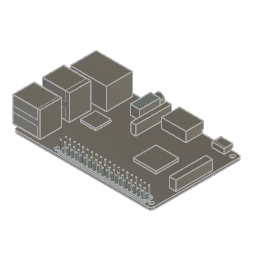
my.mesh_Gehäuse (Autodesk Fusion 360 archive; units mm, degrees)
design "Raspberry_Pi_3_B"
Autodesk Fusion 360 part; units mm, degrees
sketch "Sketch1" plane through (0, 0, 0) normal (0, 0, 1) x (1, 0, 0) in component "Pi"
  line L0 (42.5, 28) -> (-42.5, 28)
  line L1 (-42.5, 28) -> (-42.5, -28)
  line L2 (-42.5, -28) -> (42.5, -28)
  line L3 (42.5, -28) -> (42.5, 28)
  line L4 (42.5, 28) -> (-42.5, -28) construction
  line L5 (-42.5, 28) -> (42.5, -28) construction
  dimension "d1" = 85
  dimension "d2" = 56
  constraint perpendicular L0 L1
  constraint parallel L0 L2
  constraint parallel L1 L3
  constraint horizontal L0
  constraint coincident L4 origin
  constraint coincident L5 origin
  measures "d1" distance of L1.end L2.end
  measures "d2" distance of L0.end L1.end
extrude "Extrude1" add sketch "Sketch1" along normal blind 1.4 makes body 1 in component "Pi"
fillet "Fillet1" radius 2 4 edges at (42.5, -28, 0.7) (42.5, 28, 0.7) (-42.5, 28, 0.7) (-42.5, -28, 0.7) on bodies 1 in component "Pi"
sketch "Sketch2" plane through (0, 0, 1.4) normal (0, 0, 1) x (-1, 0, 0) in component "Pi"
  arc A0 (42.5, 26) -> (40.5, 28) centre (40.5, 26) ccw
  line L0 (40.5, 28) -> (-40.5, 28)
  arc A1 (-40.5, 28) -> (-42.5, 26) centre (-40.5, 26) ccw
  line L1 (-42.5, 26) -> (-42.5, -26)
  arc A2 (-42.5, -26) -> (-40.5, -28) centre (-40.5, -26) ccw
  line L2 (-40.5, -28) -> (40.5, -28)
  arc A3 (40.5, -28) -> (42.5, -26) centre (40.5, -26) ccw
  line L3 (42.5, -26) -> (42.5, 26)
  line L4 (42.5, -24.7968) -> (23.2, -24.7968) construction
  line L5 (23.2, -28) -> (23.2, -26) construction
  line L6 (23.2, -26) -> (45.5, -26)
  line L7 (45.5, -26) -> (45.5, -10)
  line L8 (45.5, -10) -> (23.2, -10)
  line L9 (23.2, -10) -> (23.2, -26)
  dimension "d6" = 19.3
  dimension "d7" = 22.3
  dimension "d8" = 16
  constraint coincident L3 L4.start
  constraint perpendicular L3 L4
  constraint coincident L2 L5.start
  constraint perpendicular L2 L5
  constraint horizontal L6
  constraint vertical L7
  constraint horizontal L8
  constraint vertical L9
  measures "d6" distance of L4.start L4.end
  measures "d7" distance of L5.end L6.end
  measures "d8" distance of L5.end L8.end
extrude "Extrude2" add sketch "Sketch2" along normal blind 13.5 contours L3 L6 L7 L8 | L3 L6 L8 L9 bodies 1 in component "Pi"
copy_body "CutPasteBodies1" bodies 1 removing the originals makes body 2 in component "Pi"
sketch "Sketch1 (1)" plane through (0, 0, 1.4) normal (0, 0, 1) x (-1, 0, 0) in component "Pi"
  line L0 (23.2, -10) -> (42.5, -10)
  line L1 (42.5, -10) -> (42.5, 26)
  arc A0 (42.5, 26) -> (40.5, 28) centre (40.5, 26) ccw
  line L2 (40.5, 28) -> (-40.5, 28)
  arc A1 (-40.5, 28) -> (-42.5, 26) centre (-40.5, 26) ccw
  line L3 (-42.5, 26) -> (-42.5, -26)
  arc A2 (-42.5, -26) -> (-40.5, -28) centre (-40.5, -26) ccw
  line L4 (-40.5, -28) -> (40.5, -28)
  arc A3 (40.5, -28) -> (42.5, -26) centre (40.5, -26) ccw
  line L5 (42.5, -26) -> (23.2, -26)
  line L6 (23.2, -26) -> (23.2, -10)
  line L7 (36, -10) -> (36, -6) construction
  line L8 (-41.9142, -27.4142) -> (-39.5808, -25.0808)
  line L9 (-41.9142, -27.4142) -> (-38.6142, -27.4142) construction
  circle A4 centre (-39.5808, -25.0808) radius 1.3
  dimension "d46" = 3.3
  dimension "d47" = 45
  dimension "d48" = 2.6
  constraint parallel L1 L7
  constraint midpoint A2 L8.start
  constraint horizontal L9
  constraint coincident L8.end A4.centre
  measures "d46" distance of L8.start L8.end
  measures "d47" angle of L8 L9
  measures "d48" diameter of A4
sketch "Sketch2 (1)" plane through (-45.5, 0, 0) normal (-1, 0, 0) x (0, -1, 0) in component "Pi"
  line L0 (-26, 1.4) -> (-10, 1.4)
  line L1 (-10, 1.4) -> (-10, 14.9)
  line L2 (-10, 14.9) -> (-26, 14.9)
  line L3 (-26, 14.9) -> (-26, 1.4)
  line L4 (-6, 1.4) -> (7.2, 1.4)
  line L5 (7.2, 1.4) -> (7.2, 17.15)
  line L6 (7.2, 17.15) -> (-6, 17.15)
  line L7 (-6, 17.15) -> (-6, 1.4)
  point P0 (-6, 1.4)
  dimension "d11" = 13.2
  dimension "d12" = 15.75
  constraint horizontal L4
  constraint vertical L5
  constraint horizontal L6
  constraint vertical L7
  constraint coincident P0 L4.start
  measures "d11" distance of P0 L4.end
  measures "d12" distance of P0 L6.end
extrude "Extrude1'" add sketch "Sketch2 (1)" against normal blind 16.7 contours L4 L5 L6 L7 bodies 2 in component "Pi"
sketch "Sketch3" plane through (-45.5, 0, 0) normal (-1, 0, 0) x (0, -1, 0) in component "Pi"
  line L0 (-6, 17.15) -> (-6, 1.4)
  line L1 (-6, 1.4) -> (7.2, 1.4)
  line L2 (7.2, 1.4) -> (7.2, 17.15)
  line L3 (7.2, 17.15) -> (-6, 17.15)
  line L4 (7.2, 1.4) -> (12.2, 1.4) construction
  line L5 (12.2, 1.4) -> (25.4, 1.4)
  line L6 (25.4, 1.4) -> (25.4, 17.15)
  line L7 (25.4, 17.15) -> (12.2, 17.15)
  line L8 (12.2, 17.15) -> (12.2, 1.4)
  dimension "d15" = 5
  dimension "d16" = 13.2
  dimension "d17" = 15.75
  constraint coincident L1.end L2.start
  constraint perpendicular L2 L4
  constraint horizontal L5
  constraint vertical L6
  constraint horizontal L7
  constraint vertical L8
  measures "d15" distance of L1.end L4.end
  measures "d16" distance of L4.end L5.end
  measures "d17" distance of L4.end L7.end
extrude "Extrude2'" add sketch "Sketch3" against normal blind 16.75 contours L5 L6 L7 L8 bodies 2 in component "Pi"
sketch "Sketch4" plane through (-45.5, 0, 0) normal (-1, 0, 0) x (0, -1, 0) in component "Pi"
  line L0 (-26, 1.4) -> (-10, 1.4)
  line L1 (-10, 1.4) -> (-10, 14.9)
  line L2 (-10, 14.9) -> (-26, 14.9)
  line L3 (-26, 14.9) -> (-26, 1.4)
  line L4 (-20.2136, 14.9) -> (-20.2136, 12.2) construction
  line L5 (-26, 12.2) -> (-24, 12.2) construction
  line L6 (-24, 12.2) -> (-12, 12.2)
  line L7 (-12, 12.2) -> (-12, 5.5)
  line L8 (-12, 5.5) -> (-24, 5.5)
  line L9 (-24, 5.5) -> (-24, 12.2)
  line L10 (-26, 5.5) -> (-21.25, 5.5) construction
  line L11 (-21.25, 5.5) -> (-15.25, 5.5)
  line L12 (-15.25, 5.5) -> (-15.25, 2)
  line L13 (-15.25, 2) -> (-21.25, 2)
  line L14 (-21.25, 2) -> (-21.25, 5.5)
  dimension "d20" = 2.7
  dimension "d21" = 12
  dimension "d22" = 6.7
  dimension "d23" = 4.75
  dimension "d24" = 6
  dimension "d25" = 3.5
  constraint coincident L2 L4.start
  constraint perpendicular L2 L4
  constraint coincident L3 L5.start
  constraint perpendicular L3 L5
  constraint horizontal L6
  constraint vertical L7
  constraint horizontal L8
  constraint vertical L9
  constraint coincident L3 L10.start
  constraint perpendicular L3 L10
  constraint horizontal L11
  constraint vertical L12
  constraint horizontal L13
  constraint vertical L14
  constraint coincident L8 L11.end
  measures "d20" distance of L4.start L4.end
  measures "d21" distance of L5.end L6.end
  measures "d22" distance of L5.end L8.end
  measures "d23" distance of L10.start L10.end
  measures "d24" distance of L10.end L11.end
  measures "d25" distance of L10.end L13.end
extrude "Extrude3" cut sketch "Sketch4" against normal blind 17 contours L6 L7 L8 L9 L11 | L8 L11 L12 L13 L14 bodies 2 in component "Pi"
sketch "Sketch5" plane through (-45.5, 0, 0) normal (-1, 0, 0) x (0, -1, 0) in component "Pi"
  line L0 (-6, 17.15) -> (-6, 1.4)
  line L1 (-6, 1.4) -> (7.2, 1.4)
  line L2 (7.2, 1.4) -> (7.2, 17.15)
  line L3 (7.2, 17.15) -> (-6, 17.15)
  line L4 (7.2, 10.975) -> (-6, 10.975)
  line L5 (-6, 10.975) -> (-6, 7.575)
  line L6 (-6, 7.575) -> (7.2, 7.575)
  line L7 (7.2, 7.575) -> (7.2, 10.975)
  line L8 (7.2, 10.975) -> (-6, 7.575) construction
  line L9 (-6, 10.975) -> (7.2, 7.575) construction
  line L10 (-5.7208, 10.975) -> (6.8067, 10.975)
  line L11 (6.8067, 10.975) -> (6.8067, 16.8566)
  line L12 (6.8067, 16.8566) -> (-5.7208, 16.8566)
  line L13 (-5.7208, 16.8566) -> (-5.7208, 10.975)
  line L14 (-5.7208, 7.6469) -> (6.8067, 7.6469)
  line L15 (6.8067, 7.6469) -> (6.8067, 1.6277)
  line L16 (6.8067, 1.6277) -> (-5.7208, 1.6277)
  line L17 (-5.7208, 1.6277) -> (-5.7208, 7.6469)
  point P0 (0.6, 9.275)
  dimension "d28" = 3.4
  constraint perpendicular L4 L5
  constraint parallel L4 L6
  constraint parallel L5 L7
  constraint horizontal L4
  constraint coincident L8 P0
  constraint coincident L9 P0
  constraint horizontal L10
  constraint vertical L11
  constraint horizontal L12
  constraint vertical L13
  constraint coincident L4 L10.start
  constraint horizontal L14
  constraint vertical L15
  constraint horizontal L16
  constraint vertical L17
  constraint coincident L8 L14.start
  measures "d28" distance of L4.end L5.end
extrude "Extrude4" cut sketch "Sketch5" against normal blind 14 contours L4 L10 L11 L12 L13 | L6 L15 L16 L17 bodies 2 in component "Pi"
sketch "Sketch6" plane through (-45.5, 0, 0) normal (-1, 0, 0) x (0, -1, 0) in component "Pi"
  line L0 (12.2, 17.15) -> (12.2, 1.4)
  line L1 (12.2, 1.4) -> (25.4, 1.4)
  line L2 (25.4, 1.4) -> (25.4, 17.15)
  line L3 (25.4, 17.15) -> (12.2, 17.15)
  line L4 (12.4971, 16.7794) -> (25.17, 16.7794)
  line L5 (25.17, 16.7794) -> (25.17, 10.9805)
  line L6 (25.17, 10.9805) -> (12.4971, 10.9805)
  line L7 (12.4971, 10.9805) -> (12.4971, 16.7794)
  line L8 (12.4971, 7.5659) -> (25.17, 7.5659)
  line L9 (25.17, 7.5659) -> (25.17, 1.5998)
  line L10 (25.17, 1.5998) -> (12.4971, 1.5998)
  line L11 (12.4971, 1.5998) -> (12.4971, 7.5659)
  constraint horizontal L4
  constraint vertical L5
  constraint horizontal L6
  constraint vertical L7
  constraint horizontal L8
  constraint vertical L9
  constraint horizontal L10
  constraint vertical L11
extrude "Extrude5" cut sketch "Sketch6" against normal blind 15 contours L4 L5 L6 L7 | L8 L9 L10 L11 bodies 2 in component "Pi"
sketch "Sketch7" plane through (0, 28, 0) normal (0, 1, 0) x (-1, 0, 0) in component "Pi"
  line L0 (40.5, 0) -> (40.5, 1.4)
  line L1 (40.5, 1.4) -> (-40.5, 1.4)
  line L2 (-40.5, 1.4) -> (-40.5, 0)
  line L3 (-40.5, 0) -> (40.5, 0)
  line L4 (42.5, 1.4) -> (42.5, 0)
  line L5 (42.5, 0.7) -> (11, 0.7) construction
  circle A0 centre (11.0002, 4.35) radius 2.95
  dimension "d33" = 31.5
  dimension "d34" = 5.9
  constraint midpoint L4 L5.start
  constraint perpendicular L0 L5
  measures "d33" distance of L5.start L5.end
  measures "d34" diameter of A0
extrude "Extrude6" add sketch "Sketch7" along normal blind 3 separate body contours A0 makes body 3 in component "Pi"
sketch "Sketch8" plane through (0, 28, 0) normal (0, -1, 0) x (1, 0, 0) in component "Pi"
  arc A0 (-10.9892, 1.4) -> (-11.0112, 1.4) centre (-11.0002, 4.35) ccw
  line L0 (-11.0112, 1.4) -> (-10.9892, 1.4)
  line L1 (-8.0502, 7.3) -> (-13.9502, 7.3)
  line L2 (-13.9502, 7.3) -> (-13.9502, 1.4)
  line L3 (-13.9502, 1.4) -> (-8.0502, 1.4)
  line L4 (-8.0502, 1.4) -> (-8.0502, 7.3)
  line L5 (-8.0502, 7.3) -> (-13.9502, 1.4) construction
  line L6 (-13.9502, 7.3) -> (-8.0502, 1.4) construction
  point P0 (-11.0002, 4.35)
  dimension "d37" = 5.9
  constraint perpendicular L1 L2
  constraint parallel L1 L3
  constraint parallel L2 L4
  constraint horizontal L1
  constraint coincident L5 P0
  constraint coincident L6 P0
  constraint coincident P0 A0.centre
  measures "d37" distance of L2.end L3.end
extrude "Extrude7" add sketch "Sketch8" along normal blind 12.5 bodies 2 3 in component "Pi"
ref_plane "WorkPlane1" through (0, 0, 1.4) normal (0, 0, 1) x (-1, 0, 0) in component "Pi"
sketch "Sketch9" plane through (0, 0, 1.4) normal (0, 0, 1) x (1, 0, 0) in component "Pi"
  line L0 (-13.9502, 15.5) -> (-13.9502, 28)
  line L1 (-28.8, 6) -> (-25.8, 6) construction
  line L2 (-25.8, 6) -> (-16.3, 6)
  line L3 (-16.3, 6) -> (-16.3, -3.5)
  line L4 (-16.3, -3.5) -> (-25.8, -3.5)
  line L5 (-25.8, -3.5) -> (-25.8, 6)
  point P0 (-28.8, 6)
  dimension "d41" = 3
  dimension "d42" = 9.5
  dimension "d43" = 9.5
  constraint coincident P0 L1.start
  constraint perpendicular L0 L1
  constraint horizontal L2
  constraint vertical L3
  constraint horizontal L4
  constraint vertical L5
  measures "d41" distance of P0 L1.end
  measures "d42" distance of L1.end L4.end
  measures "d43" distance of L1.end L2.end
extrude "Extrude8" add sketch "Sketch9" along normal blind 1.2 bodies 2 in component "Pi"
extrude "Extrude9" cut sketch "Sketch1 (1)" against normal up to surface (1.4 mm away) contours A4 bodies 2 in component "Pi"
mirror "Mirror1" about plane through (0, 0, 0) normal (0, 1, 0) of "Extrude9" in component "Pi"
sketch "Sketch10" plane through (0, 0, 1.4) normal (0, 0, 1) x (-1, 0, 0) in component "Pi"
  circle A0 centre (-39.5808, 25.0808) radius 1.3
  circle A1 centre (-39.5808, -25.0808) radius 1.3
  line L0 (25.8, 3.5) -> (25.8, -6)
  line L1 (25.8, -6) -> (16.3, -6)
  line L2 (16.3, -6) -> (16.3, 3.5)
  line L3 (16.3, 3.5) -> (25.8, 3.5)
  line L4 (13.9502, -15.5) -> (13.9502, -28)
  line L5 (13.9502, -28) -> (40.5, -28)
  arc A2 (40.5, -28) -> (42.5, -26) centre (40.5, -26) ccw
  line L6 (42.5, -26) -> (23.2, -26)
  line L7 (23.2, -26) -> (23.2, -10)
  line L8 (23.2, -10) -> (42.5, -10)
  line L9 (42.5, -10) -> (42.5, -6)
  line L10 (42.5, -6) -> (28.8, -6)
  line L11 (28.8, -6) -> (28.8, 7.2)
  line L12 (28.8, 7.2) -> (42.5, 7.2)
  line L13 (42.5, 7.2) -> (42.5, 12.2)
  line L14 (42.5, 12.2) -> (28.75, 12.2)
  line L15 (28.75, 12.2) -> (28.75, 25.4)
  line L16 (28.75, 25.4) -> (42.5, 25.4)
  line L17 (42.5, 25.4) -> (42.5, 26)
  arc A3 (42.5, 26) -> (40.5, 28) centre (40.5, 26) ccw
  line L18 (40.5, 28) -> (-40.5, 28)
  arc A4 (-40.5, 28) -> (-42.5, 26) centre (-40.5, 26) ccw
  line L19 (-42.5, 26) -> (-42.5, -26)
  arc A5 (-42.5, -26) -> (-40.5, -28) centre (-40.5, -26) ccw
  line L20 (-40.5, -28) -> (8.0502, -28)
  line L21 (8.0502, -28) -> (8.0502, -15.5)
  line L22 (8.0502, -15.5) -> (13.9502, -15.5)
  line L23 (-39.5808, 25.0808) -> (18.4192, 25.0808) construction
  circle A6 centre (18.4192, 25.0808) radius 1.35
  dimension "d52" = 58
  dimension "d53" = 2.7
  constraint coincident A0.centre L23.start
  constraint horizontal L23
  constraint coincident L23.end A6.centre
  measures "d52" distance of A0.centre L23.end
  measures "d53" diameter of A6
extrude "Extrude10" cut sketch "Sketch10" against normal up to surface (1.4 mm away) contours A6 bodies 2 in component "Pi"
mirror "Mirror2" about plane through (0, 0, 0) normal (0, 1, 0) of "Extrude10" in component "Pi"
sketch "Sketch11" plane through (0, 0, 1.4) normal (0, 0, 1) x (-1, 0, 0) in component "Pi"
  circle A0 centre (18.4192, -25.0808) radius 1.35
  circle A1 centre (18.4192, 25.0808) radius 1.35
  circle A2 centre (-39.5808, 25.0808) radius 1.3
  circle A3 centre (-39.5808, -25.0808) radius 1.3
  line L0 (25.8, 3.5) -> (25.8, -6)
  line L1 (25.8, -6) -> (16.3, -6)
  line L2 (16.3, -6) -> (16.3, 3.5)
  line L3 (16.3, 3.5) -> (25.8, 3.5)
  line L4 (13.9502, -15.5) -> (13.9502, -28)
  line L5 (13.9502, -28) -> (40.5, -28)
  arc A4 (40.5, -28) -> (42.5, -26) centre (40.5, -26) ccw
  line L6 (42.5, -26) -> (23.2, -26)
  line L7 (23.2, -26) -> (23.2, -10)
  line L8 (23.2, -10) -> (42.5, -10)
  line L9 (42.5, -10) -> (42.5, -6)
  line L10 (42.5, -6) -> (28.8, -6)
  line L11 (28.8, -6) -> (28.8, 7.2)
  line L12 (28.8, 7.2) -> (42.5, 7.2)
  line L13 (42.5, 7.2) -> (42.5, 12.2)
  line L14 (42.5, 12.2) -> (28.75, 12.2)
  line L15 (28.75, 12.2) -> (28.75, 25.4)
  line L16 (28.75, 25.4) -> (42.5, 25.4)
  line L17 (42.5, 25.4) -> (42.5, 26)
  arc A5 (42.5, 26) -> (40.5, 28) centre (40.5, 26) ccw
  line L18 (40.5, 28) -> (-40.5, 28)
  arc A6 (-40.5, 28) -> (-42.5, 26) centre (-40.5, 26) ccw
  line L19 (-42.5, 26) -> (-42.5, -26)
  arc A7 (-42.5, -26) -> (-40.5, -28) centre (-40.5, -26) ccw
  line L20 (-40.5, -28) -> (8.0502, -28)
  line L21 (8.0502, -28) -> (8.0502, -15.5)
  line L22 (8.0502, -15.5) -> (13.9502, -15.5)
  line L23 (16, 27) -> (-37.4592, 27)
  line L24 (-37.4592, 27) -> (-37.4592, 22)
  line L25 (-37.4592, 22) -> (16, 22)
  line L26 (16, 22) -> (16, 27)
  dimension "d57" = 5
  constraint horizontal L23
  constraint vertical L24
  constraint horizontal L25
  constraint vertical L26
  measures "d57" distance of L23.start L25.end
extrude "Extrude11" add sketch "Sketch11" along normal blind 1 contours L23 L24 L25 L26 bodies 2 in component "Pi"
sketch "Sketch12" plane through (0, 0, 2.4) normal (0, 0, 1) x (-1, 0, 0) in component "Pi"
  line L0 (16, 22) -> (16, 27)
  line L1 (16, 27) -> (-37.4592, 27)
  line L2 (-37.4592, 27) -> (-37.4592, 22)
  line L3 (-37.4592, 22) -> (16, 22)
  circle A0 centre (15.2841, 26.0134) radius 0.375
  dimension "d60" = 0.75
  measures "d60" diameter of A0
extrude "Extrude12" add sketch "Sketch12" along normal blind 6 contours A0 bodies 2 in component "Pi"
sketch "Sketch13" plane through (0, 0, 2.4) normal (0, 0, 1) x (-1, 0, 0) in component "Pi"
  circle A0 centre (15.2841, 26.0134) radius 0.375
  line L0 (16, 22) -> (16, 27)
  line L1 (16, 27) -> (-37.4592, 27)
  line L2 (-37.4592, 27) -> (-37.4592, 22)
  line L3 (-37.4592, 22) -> (16, 22)
ref_plane "WorkPlane2" through (10.7296, -24.5, 1.9) normal (0, -1, 0) x (1, 0, 0) in component "Pi"
mirror "Mirror3" about plane through (10.7296, -24.5, 1.9) normal (0, -1, 0) of "Extrude12" in component "Pi"
pattern_path "PathPattern2" count 20 spacing 2.7174 from (-16, -22, 1.4) along 1 edges at (10.7296, -22, 1.4) of "Extrude12", "Mirror3" on bodies 2 in component "Pi"
sketch "Sketch14" plane through (0, 0, 1.4) normal (0, 0, 1) x (-1, 0, 0) in component "Pi"
  line L0 (16, 22) -> (-37.4592, 22)
  line L1 (-37.4592, 22) -> (-37.4592, 27)
  line L2 (-37.4592, 27) -> (16, 27)
  line L3 (16, 27) -> (16, 22)
  circle A0 centre (18.4192, -25.0808) radius 1.35
  circle A1 centre (18.4192, 25.0808) radius 1.35
  circle A2 centre (-39.5808, 25.0808) radius 1.3
  circle A3 centre (-39.5808, -25.0808) radius 1.3
  line L4 (25.8, 3.5) -> (25.8, -6)
  line L5 (25.8, -6) -> (16.3, -6)
  line L6 (16.3, -6) -> (16.3, 3.5)
  line L7 (16.3, 3.5) -> (25.8, 3.5)
  line L8 (13.9502, -15.5) -> (13.9502, -28)
  line L9 (13.9502, -28) -> (40.5, -28)
  arc A4 (40.5, -28) -> (42.5, -26) centre (40.5, -26) ccw
  line L10 (42.5, -26) -> (23.2, -26)
  line L11 (23.2, -26) -> (23.2, -10)
  line L12 (23.2, -10) -> (42.5, -10)
  line L13 (42.5, -10) -> (42.5, -6)
  line L14 (42.5, -6) -> (28.8, -6)
  line L15 (28.8, -6) -> (28.8, 7.2)
  line L16 (28.8, 7.2) -> (42.5, 7.2)
  line L17 (42.5, 7.2) -> (42.5, 12.2)
  line L18 (42.5, 12.2) -> (28.75, 12.2)
  line L19 (28.75, 12.2) -> (28.75, 25.4)
  line L20 (28.75, 25.4) -> (42.5, 25.4)
  line L21 (42.5, 25.4) -> (42.5, 26)
  arc A5 (42.5, 26) -> (40.5, 28) centre (40.5, 26) ccw
  line L22 (40.5, 28) -> (-40.5, 28)
  arc A6 (-40.5, 28) -> (-42.5, 26) centre (-40.5, 26) ccw
  line L23 (-42.5, 26) -> (-42.5, -26)
  arc A7 (-42.5, -26) -> (-40.5, -28) centre (-40.5, -26) ccw
  line L24 (-40.5, -28) -> (8.0502, -28)
  line L25 (8.0502, -28) -> (8.0502, -15.5)
  line L26 (8.0502, -15.5) -> (13.9502, -15.5)
  line L27 (-42.5, 28.0113) -> (-25.5, 28.0113) construction
  line L28 (-25.5, 28.0113) -> (-25.5, 8.0113) construction
  line L29 (-25.5, 8.0113) -> (-42.5, 8.0113) construction
  line L30 (-42.5, 8.0113) -> (-42.5, 28.0113) construction
  line L31 (-25.5, 8.0113) -> (-11.5, 8.0113)
  line L32 (-11.5, 8.0113) -> (-11.5, -5.9887)
  line L33 (-11.5, -5.9887) -> (-25.5, -5.9887)
  line L34 (-25.5, -5.9887) -> (-25.5, 8.0113)
  dimension "d69" = 17
  dimension "d70" = 20
  dimension "d71" = 14
  dimension "d72" = 14
  constraint horizontal L27
  constraint vertical L28
  constraint horizontal L29
  constraint vertical L30
  constraint horizontal L31
  constraint vertical L32
  constraint horizontal L33
  constraint vertical L34
  measures "d69" distance of L27.start L27.end
  measures "d70" distance of L27.start L29.end
  measures "d71" distance of L28.end L33.end
  measures "d72" distance of L28.end L31.end
extrude "Extrude13" add sketch "Sketch14" along normal blind 1.5 contours L31 L32 L33 L34 bodies 2 in component "Pi"
sketch "Sketch15" plane through (0, 0, 7.3) normal (0, 0, 1) x (-1, 0, 0) in component "Pi"
  line L0 (8.0502, -28) -> (11.0002, -28)
  line L1 (11.0002, -28) -> (13.9502, -28)
  line L2 (13.9502, -28) -> (13.9502, -15.5)
  line L3 (13.9502, -15.5) -> (8.0502, -15.5)
  line L4 (8.0502, -15.5) -> (8.0502, -28)
sketch "Sketch16" plane through (0, 0, 1.4) normal (0, 0, 1) x (-1, 0, 0) in component "Pi"
  line L0 (-25.5, -5.9887) -> (-25.5, 8.0113)
  line L1 (-25.5, 8.0113) -> (-11.5, 8.0113)
  line L2 (-11.5, 8.0113) -> (-11.5, -5.9887)
  line L3 (-11.5, -5.9887) -> (-25.5, -5.9887)
  line L4 (16, 22) -> (-37.4592, 22)
  line L5 (-37.4592, 22) -> (-37.4592, 27)
  line L6 (-37.4592, 27) -> (16, 27)
  line L7 (16, 27) -> (16, 22)
  circle A0 centre (18.4192, -25.0808) radius 1.35
  circle A1 centre (18.4192, 25.0808) radius 1.35
  circle A2 centre (-39.5808, 25.0808) radius 1.3
  circle A3 centre (-39.5808, -25.0808) radius 1.3
  line L8 (25.8, 3.5) -> (25.8, -6)
  line L9 (25.8, -6) -> (16.3, -6)
  line L10 (16.3, -6) -> (16.3, 3.5)
  line L11 (16.3, 3.5) -> (25.8, 3.5)
  line L12 (13.9502, -15.5) -> (13.9502, -28)
  line L13 (13.9502, -28) -> (40.5, -28)
  arc A4 (40.5, -28) -> (42.5, -26) centre (40.5, -26) ccw
  line L14 (42.5, -26) -> (23.2, -26)
  line L15 (23.2, -26) -> (23.2, -10)
  line L16 (23.2, -10) -> (42.5, -10)
  line L17 (42.5, -10) -> (42.5, -6)
  line L18 (42.5, -6) -> (28.8, -6)
  line L19 (28.8, -6) -> (28.8, 7.2)
  line L20 (28.8, 7.2) -> (42.5, 7.2)
  line L21 (42.5, 7.2) -> (42.5, 12.2)
  line L22 (42.5, 12.2) -> (28.75, 12.2)
  line L23 (28.75, 12.2) -> (28.75, 25.4)
  line L24 (28.75, 25.4) -> (42.5, 25.4)
  line L25 (42.5, 25.4) -> (42.5, 26)
  arc A5 (42.5, 26) -> (40.5, 28) centre (40.5, 26) ccw
  line L26 (40.5, 28) -> (-40.5, 28)
  arc A6 (-40.5, 28) -> (-42.5, 26) centre (-40.5, 26) ccw
  line L27 (-42.5, 26) -> (-42.5, -26)
  arc A7 (-42.5, -26) -> (-40.5, -28) centre (-40.5, -26) ccw
  line L28 (-40.5, -28) -> (8.0502, -28)
  line L29 (8.0502, -28) -> (8.0502, -15.5)
  line L30 (8.0502, -15.5) -> (13.9502, -15.5)
  line L31 (8.0502, -28) -> (-2.9498, -28) construction
  line L32 (-2.9498, -28) -> (-17.9498, -28)
  line L33 (-17.9498, -28) -> (-17.9498, -18)
  line L34 (-17.9498, -18) -> (-2.9498, -18)
  line L35 (-2.9498, -18) -> (-2.9498, -28)
  dimension "d75" = 11
  dimension "d76" = 10
  dimension "d77" = 15
  constraint coincident L28.end L29.start
  constraint perpendicular L29 L31
  constraint horizontal L32
  constraint vertical L33
  constraint horizontal L34
  constraint vertical L35
  measures "d75" distance of L28.end L31.end
  measures "d76" distance of L31.end L34.end
  measures "d77" distance of L31.end L32.end
extrude "Extrude14" add sketch "Sketch16" along normal blind 6 contours L28 L32 L33 L34 L35 bodies 2 in component "Pi"
sketch "Sketch17" plane through (0, 28, 0) normal (0, 1, 0) x (-1, 0, 0) in component "Pi"
  arc A0 (8.0502, 4.35) -> (10.9892, 1.4) centre (11.0002, 4.35) ccw
  line L0 (8.0502, 4.35) -> (8.0502, 1.4)
  line L1 (8.0502, 1.4) -> (-2.9498, 1.4)
  line L2 (-2.9498, 1.4) -> (-2.9498, 7.4)
  line L3 (-2.9498, 7.4) -> (-17.9498, 7.4)
  line L4 (-17.9498, 7.4) -> (-17.9498, 1.4)
  line L5 (-17.9498, 1.4) -> (-40.5, 1.4)
  line L6 (-40.5, 1.4) -> (-40.5, 0)
  line L7 (-40.5, 0) -> (40.5, 0)
  line L8 (40.5, 0) -> (40.5, 1.4)
  line L9 (40.5, 1.4) -> (13.9502, 1.4)
  line L10 (13.9502, 1.4) -> (13.9502, 4.35)
  arc A1 (11.0112, 1.4) -> (13.9502, 4.35) centre (11.0002, 4.35) ccw
  line L11 (11.0112, 1.4) -> (10.9892, 1.4)
  line L12 (-17.9498, 7.4) -> (-2.9498, 7.4)
  line L13 (-2.9498, 7.4) -> (-2.9498, 1.4)
  line L14 (-2.9498, 1.4) -> (-17.9498, 1.4)
  line L15 (-17.9498, 1.4) -> (-17.9498, 7.4)
  constraint horizontal L12
  constraint vertical L13
  constraint horizontal L14
  constraint vertical L15
  constraint coincident L1.end L2.start
  constraint coincident L3.end L4.start
extrude "Extrude15" add sketch "Sketch17" along normal blind 1 contours L2 L3 L4 L12 L13 L14 L15 bodies 2 in component "Pi"
sketch "Sketch18" plane through (0, 0, 1.4) normal (0, 0, 1) x (-1, 0, 0) in component "Pi"
  line L0 (-17.9498, -28) -> (-17.9498, -18)
  line L1 (-17.9498, -18) -> (-2.9498, -18)
  line L2 (-2.9498, -18) -> (-2.9498, -28)
  line L3 (-2.9498, -28) -> (8.0502, -28)
  line L4 (8.0502, -28) -> (8.0502, -15.5)
  line L5 (8.0502, -15.5) -> (13.9502, -15.5)
  line L6 (13.9502, -15.5) -> (13.9502, -28)
  line L7 (13.9502, -28) -> (40.5, -28)
  arc A0 (40.5, -28) -> (42.5, -26) centre (40.5, -26) ccw
  line L8 (42.5, -26) -> (23.2, -26)
  line L9 (23.2, -26) -> (23.2, -10)
  line L10 (23.2, -10) -> (42.5, -10)
  line L11 (42.5, -10) -> (42.5, -6)
  line L12 (42.5, -6) -> (28.8, -6)
  line L13 (28.8, -6) -> (28.8, 7.2)
  line L14 (28.8, 7.2) -> (42.5, 7.2)
  line L15 (42.5, 7.2) -> (42.5, 12.2)
  line L16 (42.5, 12.2) -> (28.75, 12.2)
  line L17 (28.75, 12.2) -> (28.75, 25.4)
  line L18 (28.75, 25.4) -> (42.5, 25.4)
  line L19 (42.5, 25.4) -> (42.5, 26)
  arc A1 (42.5, 26) -> (40.5, 28) centre (40.5, 26) ccw
  line L20 (40.5, 28) -> (-40.5, 28)
  arc A2 (-40.5, 28) -> (-42.5, 26) centre (-40.5, 26) ccw
  line L21 (-42.5, 26) -> (-42.5, -26)
  arc A3 (-42.5, -26) -> (-40.5, -28) centre (-40.5, -26) ccw
  line L22 (-40.5, -28) -> (-17.9498, -28)
  line L23 (25.8, 3.5) -> (25.8, -6)
  line L24 (25.8, -6) -> (16.3, -6)
  line L25 (16.3, -6) -> (16.3, 3.5)
  line L26 (16.3, 3.5) -> (25.8, 3.5)
  circle A4 centre (-39.5808, -25.0808) radius 1.3
  circle A5 centre (-39.5808, 25.0808) radius 1.3
  circle A6 centre (18.4192, 25.0808) radius 1.35
  circle A7 centre (18.4192, -25.0808) radius 1.35
  line L27 (16, 22) -> (-37.4592, 22)
  line L28 (-37.4592, 22) -> (-37.4592, 27)
  line L29 (-37.4592, 27) -> (16, 27)
  line L30 (16, 27) -> (16, 22)
  line L31 (-25.5, -5.9887) -> (-25.5, 8.0113)
  line L32 (-25.5, 8.0113) -> (-11.5, 8.0113)
  line L33 (-11.5, 8.0113) -> (-11.5, -5.9887)
  line L34 (-11.5, -5.9887) -> (-25.5, -5.9887)
  line L35 (-41, 0) -> (-41, -11.25) construction
  line L36 (-41, -11.25) -> (-37, -11.25)
  line L37 (-37, -11.25) -> (-37, 11.25)
  line L38 (-37, 11.25) -> (-41, 11.25)
  line L39 (-41, 11.25) -> (-41, -11.25)
  dimension "d82" = 11.25
  dimension "d83" = 4
  dimension "d84" = 22.5
  constraint vertical L35
  constraint horizontal L36
  constraint vertical L37
  constraint horizontal L38
  constraint vertical L39
  measures "d82" distance of L35.start L35.end
  measures "d83" distance of L35.end L36.end
  measures "d84" distance of L35.end L38.end
extrude "Extrude16" add sketch "Sketch18" along normal blind 6 contours L36 L37 L38 L39 bodies 2 in component "Pi"
sketch "Sketch19" plane through (0, 0, 0) normal (0, 0, -1) x (1, 0, 0) in component "Pi"
  circle A0 centre (-18.4192, -25.0808) radius 1.35
  circle A1 centre (-18.4192, 25.0808) radius 1.35
  circle A2 centre (39.5808, 25.0808) radius 1.3
  circle A3 centre (39.5808, -25.0808) radius 1.3
  arc A4 (-40.5, 28) -> (-42.5, 26) centre (-40.5, 26) ccw
  line L0 (-42.5, 26) -> (-42.5, -26)
  arc A5 (-42.5, -26) -> (-40.5, -28) centre (-40.5, -26) ccw
  line L1 (-40.5, -28) -> (40.5, -28)
  arc A6 (40.5, -28) -> (42.5, -26) centre (40.5, -26) ccw
  line L2 (42.5, -26) -> (42.5, 26)
  arc A7 (42.5, 26) -> (40.5, 28) centre (40.5, 26) ccw
  line L3 (40.5, 28) -> (-40.5, 28)
  line L4 (41, -11.25) -> (41, 11.25)
  line L5 (41, 0) -> (41, 6)
  line L6 (41, 6) -> (29.5, 6)
  line L7 (29.5, 6) -> (29.5, -6)
  line L8 (29.5, -6) -> (41, -6)
  line L9 (41, -6) -> (41, 6)
  dimension "d87" = 6
  dimension "d88" = 11.5
  dimension "d89" = 12
  constraint midpoint L4 L5.start
  constraint parallel L4 L5
  constraint horizontal L6
  constraint vertical L7
  constraint horizontal L8
  constraint vertical L9
  measures "d87" distance of L5.start L5.end
  measures "d88" distance of L5.end L6.end
  measures "d89" distance of L5.end L8.end
extrude "Extrude17" add sketch "Sketch19" along normal blind 1.5 contours L4 L5 L6 L7 L8 L9 bodies 2 in component "Pi"
sketch "Sketch20" plane through (41, 0, 0) normal (1, 0, 0) x (0, 1, 0) in component "Pi"
  line L0 (6, 0) -> (-6, 0)
  line L1 (-6, 0) -> (-6, -1.5)
  line L2 (-6, -1.5) -> (6, -1.5)
  line L3 (6, -1.5) -> (6, 0)
  line L4 (-5.8, -1.3) -> (5.8, -1.3)
  line L5 (5.8, -1.3) -> (5.8, 0)
  line L6 (5.8, 0) -> (-5.8, 0)
  line L7 (-5.8, 0) -> (-5.8, -1.3)
  constraint horizontal L4
  constraint vertical L5
  constraint horizontal L6
  constraint vertical L7
extrude "Extrude18" cut sketch "Sketch20" against normal blind 10 contours L0 L4 L5 L6 L7 bodies 2 in component "Pi"
sketch "Sketch21" plane through (0, 0, 1.4) normal (0, 0, 1) x (-1, 0, 0) in component "Pi"
  line L0 (-41, 11.25) -> (-37, 11.25)
  line L1 (-37, 11.25) -> (-37, -11.25)
  line L2 (-37, -11.25) -> (-41, -11.25)
  line L3 (-41, -11.25) -> (-41, 11.25)
  line L4 (-17.9498, -28) -> (-17.9498, -18)
  line L5 (-17.9498, -18) -> (-2.9498, -18)
  line L6 (-2.9498, -18) -> (-2.9498, -28)
  line L7 (-2.9498, -28) -> (8.0502, -28)
  line L8 (8.0502, -28) -> (8.0502, -15.5)
  line L9 (8.0502, -15.5) -> (13.9502, -15.5)
  line L10 (13.9502, -15.5) -> (13.9502, -28)
  line L11 (13.9502, -28) -> (40.5, -28)
  arc A0 (40.5, -28) -> (42.5, -26) centre (40.5, -26) ccw
  line L12 (42.5, -26) -> (23.2, -26)
  line L13 (23.2, -26) -> (23.2, -10)
  line L14 (23.2, -10) -> (42.5, -10)
  line L15 (42.5, -10) -> (42.5, -6)
  line L16 (42.5, -6) -> (28.8, -6)
  line L17 (28.8, -6) -> (28.8, 7.2)
  line L18 (28.8, 7.2) -> (42.5, 7.2)
  line L19 (42.5, 7.2) -> (42.5, 12.2)
  line L20 (42.5, 12.2) -> (28.75, 12.2)
  line L21 (28.75, 12.2) -> (28.75, 25.4)
  line L22 (28.75, 25.4) -> (42.5, 25.4)
  line L23 (42.5, 25.4) -> (42.5, 26)
  arc A1 (42.5, 26) -> (40.5, 28) centre (40.5, 26) ccw
  line L24 (40.5, 28) -> (-40.5, 28)
  arc A2 (-40.5, 28) -> (-42.5, 26) centre (-40.5, 26) ccw
  line L25 (-42.5, 26) -> (-42.5, -26)
  arc A3 (-42.5, -26) -> (-40.5, -28) centre (-40.5, -26) ccw
  line L26 (-40.5, -28) -> (-17.9498, -28)
  line L27 (25.8, 3.5) -> (25.8, -6)
  line L28 (25.8, -6) -> (16.3, -6)
  line L29 (16.3, -6) -> (16.3, 3.5)
  line L30 (16.3, 3.5) -> (25.8, 3.5)
  circle A4 centre (-39.5808, -25.0808) radius 1.3
  circle A5 centre (-39.5808, 25.0808) radius 1.3
  circle A6 centre (18.4192, 25.0808) radius 1.35
  circle A7 centre (18.4192, -25.0808) radius 1.35
  line L31 (16, 22) -> (-37.4592, 22)
  line L32 (-37.4592, 22) -> (-37.4592, 27)
  line L33 (-37.4592, 27) -> (16, 27)
  line L34 (16, 27) -> (16, 22)
  line L35 (-25.5, -5.9887) -> (-25.5, 8.0113)
  line L36 (-25.5, 8.0113) -> (-11.5, 8.0113)
  line L37 (-11.5, 8.0113) -> (-11.5, -5.9887)
  line L38 (-11.5, -5.9887) -> (-25.5, -5.9887)
  line L39 (-42.5, -23.5) -> (-36, -23.5) construction
  line L40 (-36, -23.5) -> (-36, -28) construction
  line L41 (-36, -23.5) -> (-28.5, -23.5)
  line L42 (-28.5, -23.5) -> (-28.5, -28)
  line L43 (-28.5, -28) -> (-36, -28)
  line L44 (-36, -28) -> (-36, -23.5)
  dimension "d95" = 6.5
  dimension "d96" = 4.5
  dimension "d97" = 7.5
  constraint coincident L25 L39.start
  constraint perpendicular L25 L39
  constraint perpendicular L26 L40
  constraint coincident L26 L40.end
  constraint horizontal L41
  constraint vertical L42
  constraint horizontal L43
  constraint vertical L44
  measures "d95" distance of L39.start L39.end
  measures "d96" distance of L39.end L40.end
  measures "d97" distance of L39.end L41.end
extrude "Extrude19" add sketch "Sketch21" along normal blind 3 contours L26 L41 L42 L43 L44 bodies 2 in component "Pi"
sketch "Sketch22" plane through (0, 28, 0) normal (0, 1, 0) x (-1, 0, 0) in component "Pi"
  line L0 (-2.9498, 1.4) -> (-17.9498, 1.4)
  line L1 (-17.9498, 1.4) -> (-28.5, 1.4)
  line L2 (-28.5, 1.4) -> (-28.5, 4.4)
  line L3 (-28.5, 4.4) -> (-36, 4.4)
  line L4 (-36, 4.4) -> (-36, 1.4)
  line L5 (-36, 1.4) -> (-40.5, 1.4)
  line L6 (-40.5, 1.4) -> (-40.5, 0)
  line L7 (-40.5, 0) -> (40.5, 0)
  line L8 (40.5, 0) -> (40.5, 1.4)
  line L9 (40.5, 1.4) -> (13.9502, 1.4)
  line L10 (13.9502, 1.4) -> (13.9502, 4.35)
  arc A0 (11.0112, 1.4) -> (13.9502, 4.35) centre (11.0002, 4.35) ccw
  line L11 (11.0112, 1.4) -> (10.9892, 1.4)
  arc A1 (8.0502, 4.35) -> (10.9892, 1.4) centre (11.0002, 4.35) ccw
  line L12 (8.0502, 4.35) -> (8.0502, 1.4)
  line L13 (8.0502, 1.4) -> (-2.9498, 1.4)
  line L14 (-36, 4.4) -> (-28.5, 4.4)
  line L15 (-28.5, 4.4) -> (-28.5, 1.4)
  line L16 (-28.5, 1.4) -> (-36, 1.4)
  line L17 (-36, 1.4) -> (-36, 4.4)
  constraint horizontal L14
  constraint vertical L15
  constraint horizontal L16
  constraint vertical L17
  constraint coincident L1.end L2.start
  constraint coincident L3.end L4.start
extrude "Extrude20" add sketch "Sketch22" along normal blind 1 contours L2 L3 L4 L14 L15 L16 L17 bodies 2 in component "Pi"
sketch "Sketch23" plane through (0, 0, 1.4) normal (0, 0, 1) x (-1, 0, 0) in component "Pi"
  line L0 (-28.5, -23.5) -> (-28.5, -28)
  line L1 (-28.5, -28) -> (-17.9498, -28)
  line L2 (-17.9498, -28) -> (-17.9498, -18)
  line L3 (-17.9498, -18) -> (-2.9498, -18)
  line L4 (-2.9498, -18) -> (-2.9498, -28)
  line L5 (-2.9498, -28) -> (8.0502, -28)
  line L6 (8.0502, -28) -> (8.0502, -15.5)
  line L7 (8.0502, -15.5) -> (13.9502, -15.5)
  line L8 (13.9502, -15.5) -> (13.9502, -28)
  line L9 (13.9502, -28) -> (40.5, -28)
  arc A0 (40.5, -28) -> (42.5, -26) centre (40.5, -26) ccw
  line L10 (42.5, -26) -> (23.2, -26)
  line L11 (23.2, -26) -> (23.2, -10)
  line L12 (23.2, -10) -> (42.5, -10)
  line L13 (42.5, -10) -> (42.5, -6)
  line L14 (42.5, -6) -> (28.8, -6)
  line L15 (28.8, -6) -> (28.8, 7.2)
  line L16 (28.8, 7.2) -> (42.5, 7.2)
  line L17 (42.5, 7.2) -> (42.5, 12.2)
  line L18 (42.5, 12.2) -> (28.75, 12.2)
  line L19 (28.75, 12.2) -> (28.75, 25.4)
  line L20 (28.75, 25.4) -> (42.5, 25.4)
  line L21 (42.5, 25.4) -> (42.5, 26)
  arc A1 (42.5, 26) -> (40.5, 28) centre (40.5, 26) ccw
  line L22 (40.5, 28) -> (-40.5, 28)
  arc A2 (-40.5, 28) -> (-42.5, 26) centre (-40.5, 26) ccw
  line L23 (-42.5, 26) -> (-42.5, -26)
  arc A3 (-42.5, -26) -> (-40.5, -28) centre (-40.5, -26) ccw
  line L24 (-40.5, -28) -> (-36, -28)
  line L25 (-36, -28) -> (-36, -23.5)
  line L26 (-36, -23.5) -> (-28.5, -23.5)
  line L27 (-41, 11.25) -> (-37, 11.25)
  line L28 (-37, 11.25) -> (-37, -11.25)
  line L29 (-37, -11.25) -> (-41, -11.25)
  line L30 (-41, -11.25) -> (-41, 11.25)
  line L31 (25.8, 3.5) -> (25.8, -6)
  line L32 (25.8, -6) -> (16.3, -6)
  line L33 (16.3, -6) -> (16.3, 3.5)
  line L34 (16.3, 3.5) -> (25.8, 3.5)
  circle A4 centre (-39.5808, -25.0808) radius 1.3
  circle A5 centre (-39.5808, 25.0808) radius 1.3
  circle A6 centre (18.4192, 25.0808) radius 1.35
  circle A7 centre (18.4192, -25.0808) radius 1.35
  line L35 (16, 22) -> (-37.4592, 22)
  line L36 (-37.4592, 22) -> (-37.4592, 27)
  line L37 (-37.4592, 27) -> (16, 27)
  line L38 (16, 27) -> (16, 22)
  line L39 (-25.5, -5.9887) -> (-25.5, 8.0113)
  line L40 (-25.5, 8.0113) -> (-11.5, 8.0113)
  line L41 (-11.5, 8.0113) -> (-11.5, -5.9887)
  line L42 (-11.5, -5.9887) -> (-25.5, -5.9887)
  line L43 (4, -28) -> (1, -28)
  line L44 (1, -28) -> (1, -6)
  line L45 (1, -6) -> (4, -6)
  line L46 (4, -6) -> (4, -28)
  dimension "d102" = 3
  dimension "d103" = 22
  constraint horizontal L43
  constraint vertical L44
  constraint horizontal L45
  constraint vertical L46
  constraint coincident L5 L43.start
  measures "d102" distance of L43.start L43.end
  measures "d103" distance of L43.start L45.end
extrude "Extrude21" add sketch "Sketch23" along normal blind 6 contours L5 L43 L44 L45 L46 bodies 2 in component "Pi"
sketch "Sketch24" plane through (0, 31, 0) normal (0, 1, 0) x (-1, 0, 0) in component "Pi"
  arc A0 (11.0112, 1.4) -> (10.9892, 1.4) centre (11.0002, 4.35) ccw
  line L0 (10.9892, 1.4) -> (11.0112, 1.4)
  circle A1 centre (11.0002, 4.35) radius 1.75
  dimension "d106" = 3.5
  constraint concentric A0 A1
  measures "d106" diameter of A1
extrude "Extrude22" cut sketch "Sketch24" against normal blind 14 contours A1 bodies 2 in component "Pi"
sketch "Sketch25" plane through (0, 29, 0) normal (0, 1, 0) x (-1, 0, 0) in component "Pi"
  line L0 (-17.9498, 1.4) -> (-2.9498, 1.4)
  line L1 (-2.9498, 1.4) -> (-2.9498, 7.4)
  line L2 (-2.9498, 7.4) -> (-17.9498, 7.4)
  line L3 (-17.9498, 7.4) -> (-17.9498, 1.4)
  line L4 (-17.4419, 6.6859) -> (-3.5, 6.6859)
  line L5 (-3.5, 6.6859) -> (-3.5, 2)
  line L6 (-3.5, 2) -> (-17.4419, 2)
  line L7 (-17.4419, 2) -> (-17.4419, 6.6859)
  constraint horizontal L4
  constraint vertical L5
  constraint horizontal L6
  constraint vertical L7
extrude "Extrude23" cut sketch "Sketch25" against normal blind 10 contours L4 L5 L6 L7 bodies 2 in component "Pi"
chamfer "Chamfer1" distance 3 distance2 2 1 edges at (3.5, 24, 2) measured on face at (8.1473, 25.6667, 2) on bodies 2 in component "Pi"
chamfer "Chamfer2" distance 2 distance2 3 1 edges at (17.4419, 24, 2) measured on face at (17.4419, 25.6667, 3.562) on bodies 2 in component "Pi"
sketch "Sketch26" plane through (0, 29, 0) normal (0, 1, 0) x (-1, 0, 0) in component "Pi"
  line L0 (-36, 1.4) -> (-28.5, 1.4)
  line L1 (-28.5, 1.4) -> (-28.5, 4.4)
  line L2 (-28.5, 4.4) -> (-36, 4.4)
  line L3 (-36, 4.4) -> (-36, 1.4)
  line L4 (-35.5, 4) -> (-29, 4)
  line L5 (-29, 4) -> (-29, 2)
  line L6 (-29, 2) -> (-35.5, 2)
  line L7 (-35.5, 2) -> (-35.5, 4)
  constraint horizontal L4
  constraint vertical L5
  constraint horizontal L6
  constraint vertical L7
extrude "Extrude24" cut sketch "Sketch26" against normal blind 4 contours L4 L5 L6 L7 bodies 2 in component "Pi"
chamfer "Chamfer3" distance 1 distance2 2 1 edges at (35.5, 27, 2) measured on face at (35.5, 27.6667, 2.6667) on bodies 2 in component "Pi"
chamfer "Chamfer4" distance 2 distance2 1 1 edges at (29, 27, 2) measured on face at (30.5, 27.6667, 2) on bodies 2 in component "Pi"
chamfer "Chamfer5" distance 2 distance2 3 1 edges at (17.9498, 28.5, 1.4) measured on face at (17.9498, 25, 5.4) on bodies 2 in component "Pi"
chamfer "Chamfer6" distance 3 distance2 2 1 edges at (2.9498, 28.5, 1.4) measured on face at (6.9498, 28.3333, 1.4) on bodies 2 in component "Pi"
chamfer "Chamfer7" distance 1 distance2 2 1 edges at (36, 28.5, 1.4) measured on face at (36, 26.8333, 3.4) on bodies 2 in component "Pi"
chamfer "Chamfer8" distance 2 distance2 1 1 edges at (28.5, 28.5, 1.4) measured on face at (32.1667, 28.6667, 1.4) on bodies 2 in component "Pi"
component "Pi" placed x (1, 0, 0) y (0, 1, 0) z (0, 0, 1) at (0, 0, 0)
